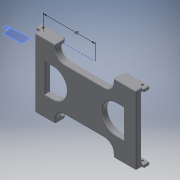
# Autodesk Inventor part: baseplate
Saved by Autodesk Inventor 2017 (Build 210142000, 142)
## iProperties
Created: 2016-08-30
Part Number: baseplate
Material: Generic
Document SubType Name: Modeling
Designer: Nic
Density: 1 g/cm^3
Appearance: Default
Author: Nic
Autodesk Inventor part; units mm, degrees
ref_plane "YZ Plane" through (0, 0, 0) normal (1, 0, 0) x (0, 1, 0)
ref_plane "XZ Plane" through (0, 0, 0) normal (0, 1, 0) x (-1, 0, 0)
ref_plane "XY Plane" through (0, 0, 0) normal (0, 0, 1) x (1, 0, 0)
sketch "Sketch2" plane through (0, 0, 0) normal (0, 0, 1) x (1, 0, 0)
  circle A0 centre (0, 0) radius 1
  line L0 (15, 2.5) -> (-3, 2.5)
  line L1 (-4, 1.5) -> (-4, -1.5)
  line L2 (-3, -2.5) -> (18, -2.5)
  line L3 (18, -2.5) -> (18, -0.5)
  line L4 (0, 0) -> (18, 0) construction
  arc A1 (-3, 2.5) -> (-4, 1.5) centre (-3, 1.5) ccw
  arc A2 (-4, -1.5) -> (-3, -2.5) centre (-3, -1.5) ccw
  arc A3 (18, -0.5) -> (15, 2.5) centre (15, -0.5) ccw
  dimension "d0" = 2
  dimension "d1" = 18
  dimension "d2" = 4
  dimension "d3" = 5
  dimension "d4" = 1
  dimension "d5" = 1
  dimension "d34" = 3
  constraints: 10 end point, 6 point on circle, 6 tangent, 4 centre point, 3 perpendicular, 2 horizontal, 1 coincident, 1 point on line, 1 other
  measures "d0" diameter of A0
  measures "d1" distance from line of L3 point (0, 0)
  measures "d2" distance from line of L1 point (0, 0)
  measures "d3" distance between parallel lines of L2 L0
  measures "d4" radius of A1
  measures "d5" radius of A2
  measures "d34" radius of A3
extrude "Extrusion1" add sketch "Sketch2" along normal blind 3
sketch "Sketch3" plane through (-3, -2.5, 0) normal (0, -1, 0) x (1, 0, 0)
  line L0 (3, 3) -> (91.2, 3)
  line L1 (91.2, 3) -> (91.2, -57)
  line L2 (91.2, -57) -> (3, -57)
  line L3 (3, -57) -> (3, 3)
  line L4 (0, 0) -> (-1, 0) construction
  line L5 (0, 0) -> (91.2, 0) construction
  line L6 (0, 0) -> (0, 3) construction
  point P0 (3, 0)
  dimension "d8" = 88.2
  dimension "d9" = 3
  dimension "d10" = 60
  dimension "d11" = 3
  constraints: 10 end point, 3 perpendicular, 1 horizontal, 1 point on line
  measures "d8" distance of L0.start L0.end
  measures "d9" distance between parallel lines of L5 L0
  measures "d10" distance between parallel lines of L2 L0
  measures "d11" distance between parallel lines of L6 L3
extrude "Extrusion2" add sketch "Sketch3" along normal blind 5
ref_plane "Work Plane1" through (44.1025, -2.5, -57) normal (-1, 0, 0) x (0, 0, 1)
mirror "Mirror1" about plane through (44.1025, -2.5, -57) normal (-1, 0, 0) of "Extrusion1"
ref_plane "Work Plane2" through (0, 0, -27) normal (0, 0, 1) x (1, 0, 0)
mirror "Mirror2" about plane through (0, 0, -27) normal (0, 0, 1) of "Extrusion1", "Mirror1"
sketch "Sketch4" plane through (-3, -7.5, 0) normal (0, -1, 0) x (1, 0, 0)
  line L0 (3, -54) -> (3, 0) projected
  line L1 (3, -27) -> (47.1025, -27) construction
  line L2 (47.1025, -27) -> (47.1025, 3.96) construction
  line L3 (3, 0) -> (21, 0) projected
  line L4 (18, 0) -> (0, 0) projected
  line L5 (3, -57) -> (91.2, -57) projected
  line L6 (27.9512, -4.04) -> (66.2538, -4.04)
  arc A0 (21, 0) -> (27.9512, -4.04) centre (27.9512, 3.96) ccw
  arc A1 (66.2538, -4.04) -> (73.205, 0) centre (66.2538, 3.96) ccw
  line L7 (21, 0) -> (18, 0) projected
  line L8 (21, 0) -> (21, 15.96)
  line L9 (21, 15.96) -> (73.205, 15.96)
  line L10 (73.205, 15.96) -> (73.205, 0)
  line L11 (12, -15) -> (12, -27)
  line L12 (12, -15) -> (18.5, -15)
  arc A2 (30.5, -27) -> (18.5, -15) centre (18.5, -27) ccw
  line L13 (12, -27) -> (12, -39)
  line L14 (12, -39) -> (18.5, -39)
  arc A3 (18.5, -39) -> (30.5, -27) centre (18.5, -27) ccw
  line L15 (27.9512, -49.96) -> (66.2538, -49.96)
  arc A4 (27.9512, -49.96) -> (21, -54) centre (27.9512, -57.96) ccw
  arc A5 (73.205, -54) -> (66.2538, -49.96) centre (66.2538, -57.96) ccw
  line L16 (21, -54) -> (21, -69.96)
  line L17 (21, -69.96) -> (73.205, -69.96)
  line L18 (73.205, -69.96) -> (73.205, -54)
  line L19 (82.205, -15) -> (82.205, -27)
  line L20 (82.205, -15) -> (75.705, -15)
  arc A6 (75.705, -15) -> (63.705, -27) centre (75.705, -27) ccw
  line L21 (82.205, -27) -> (82.205, -39)
  line L22 (82.205, -39) -> (75.705, -39)
  arc A7 (63.705, -27) -> (75.705, -39) centre (75.705, -27) ccw
  point P0 (20, 0)
  dimension "d16" = 44.1025
  dimension "d48" = 8
  dimension "d49" = 16
  dimension "d51" = 52.205
  dimension "d52" = 12
  dimension "d54" = 9
  dimension "d55" = 12
  dimension "d56" = 12
  dimension "d57" = 6.5
  dimension "d60" = 38.3027
  constraints: 38 end point, 18 point on circle, 18 symmetric about line, 8 centre point, 4 perpendicular, 4 tangent, 3 vertical, 2 horizontal, 2 point on line, 1 collinear, 1 midpoint, 6 other
  measures "d16" distance of L1.start L1.end
  measures "d48" distance from line of L2.end L6
  measures "d49" diameter of A0
  measures "d51" distance between parallel lines of L8 L10
  measures "d52" distance from line of A0.centre L9
  measures "d54" distance between parallel lines of L0 L11
  measures "d55" radius of A2
  measures "d56" distance between parallel lines of L1 L12
  measures "d57" distance from line of L11 A2.centre
  measures "d60" distance of A1.centre A0.centre
extrude "Extrusion3" cut sketch "Sketch4" along normal through all both and the other way through all
fillet "Fillet6" radius 1 52 edges at (9, -7.5, 3) (79.2025, -7.5, 3) (-3.7071, 2.2071, 3) (-4, 0, 3) (-3.7071, -2.2071, 3) (-1.5, -2.5, 3) (17.1213, 1.6213, 3) (71.0837, 1.6213, 3) (82.205, 2.5, 3) (91.9121, 2.2071, 3) (92.205, 0, 3) (91.9121, -2.2071, 3) (89.7025, -2.5, 3) (6, 2.5, 3) (-3.7071, 2.2071, 0) (-4, 0, 0) (-3.7071, -2.2071, 0) (-1.5, -2.5, 0) (17.1213, 1.6213, 0) (6, 2.5, 0) (89.7025, -2.5, -57) (-1.5, -2.5, -57) (17.1213, 1.6213, -57) (6, 2.5, -57) (-3.7071, 2.2071, -57) (-4, 0, -57) (-3.7071, -2.2071, -57) (71.0837, 1.6213, -57) (82.205, 2.5, -57) (91.9121, 2.2071, -57) (92.205, 0, -57) (91.9121, -2.2071, -57) (79.2025, -7.5, -57) (9, -7.5, -57) (91.9121, -2.2071, -54) (89.7025, -2.5, -54) (91.9121, 2.2071, -54) (82.205, 2.5, -54) (71.0837, 1.6213, -54) (92.205, 0, -54) (-3.7071, -2.2071, -54) (-1.5, -2.5, -54) (-3.7071, 2.2071, -54) (6, 2.5, -54) (17.1213, 1.6213, -54) (-4, 0, -54) (91.9121, 2.2071, 0) (92.205, 0, 0) (91.9121, -2.2071, 0) (89.7025, -2.5, 0) (71.0837, 1.6213, 0) (82.205, 2.5, 0)
fillet "Fillet7" radius 1 1 edges at (79.7025, -2.5, 0)
fillet "Fillet8" radius 1 3 edges at (8.5, -2.5, 0) (8.5, -2.5, -54) (79.7025, -2.5, -54)
fillet "Fillet9" radius 0.5 46 edges at (70.4979, -7.2071, -56.7071) (67.4632, -7.5, -51.1569) (44.1025, -7.5, -49.96) (20.7418, -7.5, -51.1569) (18, -7.5, -55.5) (17.7071, -7.2071, -56.7071) (70.205, -7.5, -55.5) (88.2, -2.2071, -53.7071) (88.2, -2.2071, -0.2929) (88.2, -2.5, -27) (79.205, -2.5, -27) (75.955, -2.5, -39) (75.955, -2.5, -15) (60.705, -2.5, -27) (12.25, -2.5, -15) (12.25, -2.5, -39) (27.5, -2.5, -27) (9, -2.5, -27) (0, -2.2071, -0.2929) (0, -2.2071, -53.7071) (0, -2.5, -27) (0, -7.2071, -56.7071) (0, -4, -57) (0, -7.2071, 2.7071) (0, -4, 3) (0, -7.5, -27) (44.1025, -7.5, -4.04) (20.7418, -7.5, -2.8431) (18, -7.5, 1.5) (17.7071, -7.2071, 2.7071) (70.205, -7.5, 1.5) (70.4979, -7.2071, 2.7071) (67.4632, -7.5, -2.8431) (9, -7.5, -27) (12.25, -7.5, -39) (12.25, -7.5, -15) (27.5, -7.5, -27) (75.955, -7.5, -15) (75.955, -7.5, -39) (60.705, -7.5, -27) (79.205, -7.5, -27) (88.2, -7.2071, 2.7071) (88.2, -4, 3) (88.2, -7.2071, -56.7071) (88.2, -4, -57) (88.2, -7.5, -27)
sketch "Sketch7" plane through (0, 0, 0) normal (0, 1, 0) x (-1, 0, 0)
  line L0 (0, 0) -> (-45, 0) construction
  dimension "d59" = 45
  constraints: 2 end point, 1 horizontal
  measures "d59" distance of L0.start L0.end
body "Solid1"
